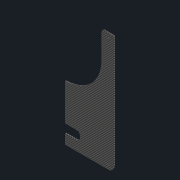
# Autodesk Inventor part: base7
Saved by Autodesk Inventor 2021 (Build 250183000, 183)
## iProperties
Created: 2021-07-20
Part Number: base7
Material: CFRP
Document SubType Name: Sheet Metal
Designer: yuta0
Density: 1.43 g/cm^3
Sheet Metal Rule: Default_mm
Appearance: カーボンファイバー
Author: yuta0
Autodesk Inventor part; units mm, degrees
ref_plane "XZ Plane" through (0, 0, 0) normal (0, 1, 0) x (-1, 0, 0)
ref_plane "XY Plane" through (0, 0, 0) normal (0, 0, 1) x (1, 0, 0)
sketch "スケッチ2" plane through (0, 0, 2) normal (0, 0, 1) x (1, 0, 0)
  circle A0 centre (0, 0) radius 44.5
  dimension "d5" = 89
  constraints: 1 centre point, 1 coincident
  measures "d5" diameter of A0
sketch "スケッチ1" plane through (0, 0, 0) normal (0, 0, 1) x (1, 0, 0)
  line L0 (-90, -170) -> (90, -170)
  line L1 (90, -170) -> (90, 70)
  line L2 (90, 70) -> (-90, 70)
  line L3 (-90, 70) -> (-90, -170)
  point P0 (0, 0)
  point P1 (-29.0861, -170)
  dimension "d37" = 90
  dimension "d38" = 70
  dimension "d40" = 90
  dimension "d41" = 170
  constraints: 8 end point, 2 parallel, 1 horizontal, 1 perpendicular, 1 point on line
  measures "d37" distance from line of L1 point (0, 0)
  measures "d38" distance from line of point (0, 0) L2
  measures "d40" distance from line of point (0, 0) L3
  measures "d41" distance from line of point (0, 0) L0
extrude "プレート1" add sketch "スケッチ1" along normal blind 2
extrude "押し出し1" cut sketch "スケッチ2" against normal blind 10
sketch "スケッチ3" plane through (0, 0, 2) normal (0, 0, 1) x (1, 0, 0)
  circle A0 centre (0, 0) radius 62.5
  point P0 (-16.1762, 60.3704)
  point P1 (-44.1942, 44.1942)
  point P2 (-60.3704, 16.1762)
  point P3 (-60.3704, -16.1762)
  point P4 (-44.1942, -44.1942)
  point P5 (-16.1762, -60.3704)
  point P6 (16.1762, -60.3704)
  point P7 (44.1942, -44.1942)
  point P8 (60.3704, -16.1762)
  point P9 (60.3704, 16.1762)
  point P10 (44.1942, 44.1942)
  point P11 (16.1762, 60.3704)
  dimension "d8" = 125
  dimension "d11" = 360
  dimension "d20" = 0
  constraints: 1 coincident, 16 other
  measures "d20" vertical distance of point (16.176, 60.37) point (-16.176, 60.37)
hole "穴1" at (-16.1762, 60.3704, 2) at (-44.1942, 44.1942, 2) at (-60.3704, 16.1762, 2) at (-60.3704, -16.1762, 2) at (-44.1942, -44.1942, 2) at (-16.1762, -60.3704, 2) at (16.1762, -60.3704, 2) at (44.1942, -44.1942, 2) at (60.3704, -16.1762, 2) at (60.3704, 16.1762, 2) at (44.1942, 44.1942, 2) at (16.1762, 60.3704, 2) direction (0, 0, -1) diameter 4.5 end through all clearance for "Flat Head Machine Screw" size "M4" standard "Ansi Metric M Profile"
fillet "コーナーR2" radius 10 4 edges at (-90, 70, 1) (90, 70, 1) (90, -170, 1) (-90, -170, 1)
sketch "スケッチ5" plane through (0, 0, 2) normal (0, 0, 1) x (1, 0, 0)
  arc A0 (-80, 70) -> (-90, 60) centre (-80, 60) ccw projected
  arc A1 (90, 60) -> (80, 70) centre (80, 60) ccw projected
  arc A2 (-90, -160) -> (-80, -170) centre (-80, -160) ccw projected
  arc A3 (80, -170) -> (90, -160) centre (80, -160) ccw projected
  point P0 (0, 0)
hole "穴2" at (-80, 60, 2) at (80, 60, 2) at (-80, -160, 2) at (80, -160, 2) direction (0, 0, -1) diameter 3.4 end through all clearance for "Socket Head Cap Screw" size "M3" standard "Ansi Metric M Profile"
sketch "スケッチ7" plane through (0, 0, 2) normal (0, 0, 1) x (1, 0, 0)
  circle A0 centre (0, 0) radius 44.5 projected
  circle A1 centre (0, 0) radius 67.5
  line L0 (90, -170) -> (-90, -170) projected
  line L1 (-90, -170) -> (-90, 60) projected
  line L2 (-90, -170) -> (-67.5, -170)
  line L3 (-67.5, -170) -> (-67.5, 50)
  line L4 (-67.5, 50) -> (-90, 50)
  line L5 (-90, 50) -> (-90, -170)
  line L6 (90, -170) -> (67.5, -170)
  line L7 (67.5, -170) -> (67.5, 50)
  line L8 (67.5, 50) -> (90, 50)
  line L9 (90, 50) -> (90, -170)
  line L10 (-80, 70) -> (80, 70) projected
  arc A2 (-80, 70) -> (-90, 60) centre (-80, 60) ccw projected
  arc A3 (90, 60) -> (80, 70) centre (80, 60) ccw projected
  line L11 (90, 60) -> (90, -170) projected
  point P0 (67.5, 0)
  point P1 (0, -173)
  point P2 (-67.5, 0)
  point P3 (-67.5, -170)
  dimension "d56" = 20
  dimension "d57" = 20
  dimension "d76" = 135
  constraints: 16 end point, 4 parallel, 2 horizontal, 2 perpendicular, 2 tangent, 1 centre point, 1 coincident
  measures "d56" distance between parallel lines of L10 L4
  measures "d57" distance between parallel lines of L10 L8
  measures "d76" diameter of A1
extrude "押し出し4" cut sketch "スケッチ7" against normal blind 10 contours A0 | A1 | A1 L3 L4 L1 A2 L10 A3 L11 L8 L7
fillet "コーナーR4" radius 5 2 edges at (-67.5, 50, 1) (67.5, 50, 1)
sketch "スケッチ8" plane through (0, 0, 2) normal (0, 0, 1) x (1, 0, 0)
  line L0 (90, -170) -> (-90, -170) projected
  line L1 (-20, -143.8) -> (20, -143.8) construction
  line L2 (-20, -153.8) -> (20, -153.8)
  line L3 (20, -133.8) -> (-20, -133.8)
  arc A0 (-20, -133.8) -> (-20, -153.8) centre (-20, -143.8) ccw
  arc A1 (20, -153.8) -> (20, -133.8) centre (20, -143.8) ccw
  point P0 (0, 0)
  point P1 (0, -143.8)
  dimension "d73" = 26.2
  dimension "d74" = 40
  dimension "d75" = 10
  constraints: 8 end point, 4 point on circle, 4 tangent, 2 centre point, 1 midpoint, 1 parallel, 1 vertical alignment
  measures "d73" distance between parallel lines of L0 L1
  measures "d74" distance of L1.end L1.start
  measures "d75" radius of A1
extrude "押し出し5" cut sketch "スケッチ8" against normal blind 10
sketch "スケッチ9" plane through (0, 0, 2) normal (0, 0, 1) x (1, 0, 0)
  circle A0 centre (-80, -160) radius 1.7 projected
  circle A1 centre (80, -160) radius 1.7 projected
  line L0 (90, 50) -> (72.5, 50) projected
  point P0 (0, 0)
  point P1 (-80, 40)
  point P2 (80, 40)
  dimension "d65" = 10
  constraints: 2 vertical alignment, 1 horizontal alignment
  measures "d65" distance from line of L0 point (80, 40)
hole "穴3" at (-80, 40, 2) at (80, 40, 2) direction (0, 0, -1) diameter 3.4 end through all clearance for "Socket Head Cap Screw" size "M3" standard "Ansi Metric M Profile"
split "スカルプ1" plane through (0, 0, 0) removes the side toward (-1, 0, 0)
equation "\"d40\" = d37"
equation "\"d18\" = Thickness"
equation "\"d47\" = Thickness"
equation "\"d71\" = Thickness"
equation "\"d2\" = Thickness"
equation "\"BendRadius\" = Thickness"
equation "\"BendReliefWidth\" = Thickness"
equation "\"BendReliefDepth\" = 0.5 * Thickness"
equation "\"CornerReliefSize\" = 4 * Thickness"
equation "\"MinimumRemnant\" = 2 * Thickness"
equation "\"TransitionRadius\" = BendRadius"
equation "\"JacobiRadiusSize\" = BendRadius"
equation "\"GapSize\" = Thickness"
equation "\"Thickness\" = 2"
